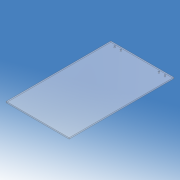
# Autodesk Inventor part: NASA-20-EBOX-LID-REV1-01
Saved by Autodesk Inventor 2020 (Build 240168000, 168)
## iProperties
Created: 2019-09-23
Part Number: NASA-20-EBOX-LID-REV1-01
Material: Polycarbonate, Smoke
Document SubType Name: Modeling
Designer: mpark
Density: 1.2 g/cm^3
Appearance: Polycarbonate - Clear
Mass: 184.217 g
Surface Area: 996.201 cm^2
Volume: 153.514 cm^3
Author: mpark
Title: Electronics Box Lid
Autodesk Inventor part; units mm, degrees
ref_plane "YZ Plane" through (0, 0, 0) normal (1, 0, 0) x (0, 1, 0)
ref_plane "XZ Plane" through (0, 0, 0) normal (0, 1, 0) x (-1, 0, 0)
ref_plane "XY Plane" through (0, 0, 0) normal (0, 0, 1) x (1, 0, 0)
sketch "Sketch1" plane through (0, 0, 0) normal (0, 1, 0) x (-1, 0, 0)
  line L0 (81.55, 135.525) -> (-81.55, 135.525)
  line L1 (-81.55, 135.525) -> (-81.55, -135.525)
  line L2 (-81.55, -135.525) -> (81.55, -135.525)
  line L3 (81.55, -135.525) -> (81.55, 135.525)
  line L4 (81.55, 135.525) -> (-81.55, -135.525) construction
  line L5 (-81.55, 135.525) -> (81.55, -135.525) construction
  point P0 (0, 0)
  dimension "d0" = 163.1
  dimension "d1" = 271.05
  constraints: 12 end point, 2 midpoint, 2 parallel, 1 horizontal, 1 perpendicular
  measures "d0" distance of L2.end L1.end
  measures "d1" distance of L1.end L0.end
extrude "Extrusion1" add sketch "Sketch1" along normal blind 3.175
sketch "Sketch2" plane through (0, 3.175, 0) normal (0, 1, 0) x (1, 0, 0)
  line L0 (81.55, 135.525) -> (-81.55, 135.525) projected
  line L1 (-81.55, 135.525) -> (-81.55, -135.525) projected
  line L2 (-81.55, -135.525) -> (81.55, -135.525) projected
  line L3 (81.55, -135.525) -> (81.55, 135.525) projected
  line L4 (-49.1236, 135.0962) -> (-54.7878, 135.0962) projected
  line L5 (-54.7878, 135.0962) -> (-54.7878, 136.525) projected
  line L6 (-59.5122, 136.525) -> (-54.7878, 136.525) projected
  line L7 (-59.5122, 136.525) -> (-59.5122, 135.0962) projected
  line L8 (-59.5122, 135.0962) -> (-65.1764, 135.0962) projected
  line L9 (-65.1764, 135.0962) -> (-65.1764, 136.525) projected
  line L10 (-69.85, 136.525) -> (-65.1764, 136.525) projected
  line L11 (-69.85, 123.825) -> (-69.85, 136.525) projected
  line L12 (-69.85, 123.825) -> (-44.45, 123.825) projected
  line L13 (-44.45, 123.825) -> (-44.45, 136.525) projected
  line L14 (-49.1236, 136.525) -> (-44.45, 136.525) projected
  line L15 (-49.1236, 136.525) -> (-49.1236, 135.0962) projected
  circle A0 centre (-49.2125, 128.9844) radius 2.0955 projected
  circle A1 centre (-65.0875, 128.9844) radius 2.0955 projected
  line L16 (65.1764, 135.0962) -> (59.5122, 135.0962) projected
  line L17 (59.5122, 135.0962) -> (59.5122, 136.525) projected
  line L18 (54.7878, 136.525) -> (59.5122, 136.525) projected
  line L19 (54.7878, 136.525) -> (54.7878, 135.0962) projected
  line L20 (54.7878, 135.0962) -> (49.1236, 135.0962) projected
  line L21 (49.1236, 135.0962) -> (49.1236, 136.525) projected
  line L22 (44.45, 136.525) -> (49.1236, 136.525) projected
  line L23 (44.45, 123.825) -> (44.45, 136.525) projected
  line L24 (44.45, 123.825) -> (69.85, 123.825) projected
  line L25 (69.85, 123.825) -> (69.85, 136.525) projected
  line L26 (65.1764, 136.525) -> (69.85, 136.525) projected
  line L27 (65.1764, 136.525) -> (65.1764, 135.0962) projected
  circle A2 centre (65.0875, 128.9844) radius 2.0955 projected
  circle A3 centre (49.2125, 128.9844) radius 2.0955 projected
  point P0 (0, 0)
hole "Hole1" at (-49.2125, 3.175, -128.9844) at (-65.0875, 3.175, -128.9844) at (49.2125, 3.175, -128.9844) at (65.0875, 3.175, -128.9844) direction (0, -1, 0) diameter 3.5 end through all
body "Solid1"
